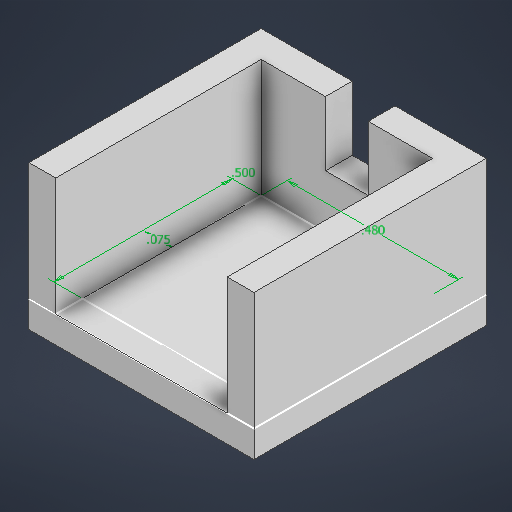
# Autodesk Inventor part: SolenoidHolder
Saved by Autodesk Inventor 2026.2 (Build 302298010, 298A)
## iProperties
Created: 2026-03-08
Part Number: SolenoidHolder
Material: Generic
Document SubType Name: Modeling
Designer: david
Density: 1 g/cm^3
Appearance: Default
Author: david
Autodesk Inventor part; units mm, degrees
ref_plane "YZ Plane" through (0, 0, 0) normal (1, 0, 0) x (0, 1, 0)
ref_plane "XZ Plane" through (0, 0, 0) normal (0, 1, 0) x (-1, 0, 0)
ref_plane "XY Plane" through (0, 0, 0) normal (0, 0, 1) x (1, 0, 0)
sketch "Sketch1" plane through (0, 0, 0) normal (0, 1, 0) x (-1, 0, 0)
  line L0 (0, 0) -> (12.192, 0)
  line L1 (12.192, 0) -> (12.192, -12.7)
  line L2 (12.192, -12.7) -> (0, -12.7)
  line L3 (0, -12.7) -> (0, 0)
  line L4 (14.097, -14.605) -> (14.097, 1.905)
  line L5 (14.097, 1.905) -> (-1.905, 1.905)
  line L6 (-1.905, 1.905) -> (-1.905, -14.605)
  line L7 (-1.905, -14.605) -> (14.097, -14.605)
  line L8 (12.192, 0) -> (12.192, 1.905)
  line L9 (0, 0) -> (0, 1.905)
  dimension "d0" = 12.192
  dimension "d1" = 12.7
  dimension "d2" = 1.905
  constraints: 20 end point, 4 parallel, 3 perpendicular, 2 point on line, 1 horizontal, 1 vertical, 3 other
  measures "d0" distance of L1.end L2.end
  measures "d1" distance of L0.end L1.end
  measures "d2" distance between parallel lines of L1 L4
extrude "Extrusion1" add sketch "Sketch1" along normal blind 8.382 contours L3 L2 L1 L8 L5 L4 L7 L6 L9
extrude "Extrusion2" add sketch "Sketch1" against normal blind 1.905
sketch "Sketch2" plane through (0, -1.905, 0) normal (0, -1, 0) x (1, 0, 0)
  circle A0 centre (-6.096, -4.4663) radius 3.7846
  line L0 (-14.097, 1.905) -> (-14.097, -14.605) projected
  point P0 (0, 0)
  dimension "d7" = 7.5692
  dimension "d8" = 8.001
  constraints: 1 centre point
  measures "d7" diameter of A0
  measures "d8" distance from line of L0 A0.centre
extrude "Extrusion3" add sketch "Sketch2" along normal blind 1.905
sketch "Sketch3" plane through (1.905, 8.382, -14.605) normal (0, 0, -1) x (-1, 0, 0)
  line L0 (0, 0) -> (16.002, 0) projected
  line L1 (6.477, 0) -> (9.525, 0)
  line L2 (9.525, 0) -> (9.525, -4.572)
  line L3 (9.525, -4.572) -> (6.477, -4.572)
  line L4 (6.477, -4.572) -> (6.477, 0)
  line L5 (14.097, -8.382) -> (1.905, -8.382) projected
  line L6 (0, -10.287) -> (0, 0) projected
  line L7 (1.905, -8.382) -> (1.905, 0) projected
  dimension "d11" = 3.81
  dimension "d13" = 3.048
  dimension "d14" = 4.572
  constraints: 8 end point, 2 parallel, 1 horizontal, 1 perpendicular, 1 point on line
  measures "d11" distance between parallel lines of L5 L3
  measures "d13" distance between parallel lines of L4 L2
  measures "d14" distance between parallel lines of L4 L7
extrude "Extrusion4" cut sketch "Sketch3" against normal blind 1.905
body "Solid1"
